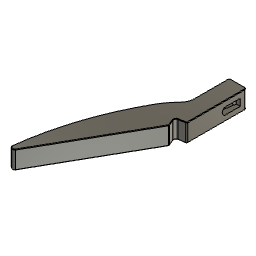
MitiVac Handle v3 (Autodesk Fusion 360 design; units mm, degrees)
Autodesk Fusion 360 part; units mm, degrees
sketch "Sketch1" plane through (0, 0, 0) normal (1, 0, 0) x (0, 1, 0) in component "MitiVac Handle"
  line L0 (0, 0) -> (0, 3.5)
  line L1 (0, 3.5) -> (53.5, 3.5)
  line L2 (53.5, 3.5) -> (53.5, 0)
  line L3 (53.5, 0) -> (37.5, 0)
  line L4 (37.5, 0) -> (35.5, 0)
  line L5 (37.5, 0) -> (37.5, 3.5)
  line L6 (0, 0) -> (0, -3.5)
  line L7 (0, -3.5) -> (53.5, -3.5)
  line L8 (53.5, -3.5) -> (53.5, 0)
  line L9 (37.5, 0) -> (37.5, -3.5)
  arc A0 (37.5, 3.5) -> (37.5, -3.5) centre (39.5625, 0) ccw
  line L10 (0, 0) -> (53.5, 0)
  line L11 (0, 0) -> (53.5, 0)
  line L12 (0, 3.5) -> (0, 9)
  line L13 (0, -3.5) -> (0, -9)
  line L14 (0, 9) -> (30, 9)
  line L15 (30, 9) -> (30, 12.5)
  line L16 (30, 12.5) -> (60, 12.5)
  line L17 (60, 12.5) -> (60, 0)
  line L18 (0, -9) -> (30, -9)
  line L19 (30, -9) -> (30, -12.5)
  line L20 (30, -12.5) -> (60, -12.5)
  line L21 (60, -12.5) -> (60, 0)
  dimension "d1" = 3.5
  dimension "d2" = 53.5
  dimension "d3" = 3.5
  dimension "d4" = 16
  dimension "d5" = 2
  dimension "d6" = 3.5
  dimension "d7" = 53.5
  dimension "d8" = 5.5
  dimension "d9" = 5.5
  dimension "d10" = 30
  dimension "d11" = 3.5
  dimension "d12" = 30
  dimension "d13" = 12.5
  dimension "d14" = 30
  dimension "d15" = 3.5
  dimension "d16" = 30
  constraint coincident L0.start L6.start
  constraint vertical L0
  constraint perpendicular L0 L1
  constraint perpendicular L1 L2
  constraint perpendicular L2 L3
  constraint parallel L3 L4
  constraint coincident L1 L5.end
  constraint perpendicular L1 L5
  constraint parallel L0 L6
  constraint perpendicular L6 L7
  constraint coincident L7 L9.end
  constraint perpendicular L7 L9
  constraint coincident L4.end A0
  constraint perpendicular L1 L12
  constraint perpendicular L7 L13
  constraint perpendicular L12 L14
  constraint perpendicular L14 L15
  constraint perpendicular L15 L16
  constraint perpendicular L16 L17
  constraint perpendicular L13 L18
  constraint perpendicular L18 L19
  constraint perpendicular L19 L20
  measures "d1" distance of L0.start L0.end
  measures "d2" distance of L0.end L1.end
  measures "d3" distance of L1.end L2.end
  measures "d4" distance of L2.end L3.end
  measures "d5" distance of L3.end L4.end
  measures "d6" distance of L0.start L6.end
  measures "d7" distance of L6.end L7.end
  measures "d8" distance of L0.end L12.end
  measures "d9" distance of L6.end L13.end
  measures "d10" distance of L12.end L14.end
  measures "d11" distance of L14.end L15.end
  measures "d12" distance of L15.end L16.end
  measures "d13" distance of L16.end L17.end
  measures "d14" distance of L13.end L18.end
  measures "d15" distance of L18.end L19.end
  measures "d16" distance of L19.end L20.end
sketch "Sketch2" plane through (0, 0, 0) normal (0, 0, 1) x (1, 0, 0) in component "MitiVac Handle"
  line L0 (0, 0) -> (0, 53.5)
  line L1 (0, 0) -> (-10.667, -1.6895)
  line L2 (0, 0) -> (9, 0) construction
  line L3 (-10.667, -1.6895) -> (-6.7597, -10.8945)
  line L4 (-10.667, -1.6895) -> (-0.667, -1.6895) construction
  line L5 (0, 0) -> (-6.7597, -10.8945)
  line L6 (-6.7597, -10.8945) -> (18.2403, -10.8945) construction
  line L7 (0, 0) -> (0, -40)
  line L8 (0, -40) -> (-63.5674, -110.5988)
  line L9 (0, -40) -> (95, -40) construction
  line L10 (-63.5674, -110.5988) -> (-6.7597, -10.8945)
  line L11 (0, 53.5) -> (0, 60)
  line L12 (0, 60) -> (-12.5, 60)
  line L13 (-12.5, 60) -> (-12.5, 25)
  line L14 (-63.5674, -110.5988) -> (-67.9117, -108.1235)
  line L15 (-10.667, -1.6895) -> (-28.7932, 6.7629)
  line L16 (-10.667, -1.6895) -> (9.333, -1.6895) construction
  line L17 (-28.7932, 6.7629) -> (-12.5, 25)
  line L18 (-28.7932, 6.7629) -> (-54.1503, -47.6156)
  arc A0 (-28.7932, 6.7629) -> (-67.9117, -108.1235) centre (217.624, -141.2447) ccw
  line L19 (0, 53.5) -> (-4, 53.5)
  line L20 (0, 53.5) -> (0, 37.5)
  line L21 (0, 37.5) -> (0, 35.5)
  line L22 (0, 37.5) -> (-6.5, 37.5)
  line L23 (-6.5, 37.5) -> (-4, 53.5)
  line L24 (-12.5, 60) -> (-12.5, 56)
  line L25 (-12.5, 56) -> (-4, 53.5)
  line L26 (-6.5, 37.5) -> (-12.5, 37.5)
  line L27 (-12.5, 37.5) -> (-12.5, 35.5)
  line L28 (-6.5, 37.5) -> (-12.5, 35.5)
  line L29 (-12.5, 60) -> (-17.5, 60)
  line L30 (-17.5, 60) -> (-17.5, 19.4035)
  line L31 (-12.5, 35.5) -> (-17.5, 33.8333)
  line L32 (-12.5, 56) -> (-17.5, 57.4706)
  dimension "d17" = 53.5
  dimension "d18" = 10.8
  dimension "d19" = 171
  dimension "d20" = 67
  dimension "d21" = 10
  dimension "d24" = 40
  dimension "d25" = 132
  dimension "d26" = 95
  dimension "d27" = 6.5
  dimension "d28" = 12.5
  dimension "d29" = 35
  dimension "d30" = 5
  dimension "d31" = 155
  dimension "d32" = 20
  dimension "d33" = 60
  dimension "d34" = 4
  dimension "d35" = 16
  dimension "d36" = 2
  dimension "d37" = 6.5
  dimension "d38" = 4
  dimension "d39" = 2
  dimension "d66" = 5
  constraint coincident L0.start L1.start
  constraint vertical L0
  constraint horizontal L2
  constraint horizontal L4
  constraint horizontal L6
  constraint perpendicular L6 L7
  constraint horizontal L9
  constraint parallel L0 L11
  constraint perpendicular L11 L12
  constraint perpendicular L12 L13
  constraint perpendicular L10 L14
  constraint horizontal L16
  constraint perpendicular L15 L18
  constraint coincident L18.end A0
  constraint perpendicular L0 L19
  constraint coincident L0 L20.end
  constraint parallel L0 L21
  constraint perpendicular L20 L22
  constraint perpendicular L19 L24
  constraint coincident L13 L26.end
  constraint perpendicular L13 L26
  constraint perpendicular L26 L27
  constraint perpendicular L24 L29
  constraint coincident L17 L30.end
  constraint perpendicular L29 L30
  constraint coincident L30 L31.end
  constraint parallel L28 L31
  constraint coincident L30 L32.end
  constraint parallel L25 L32
  measures "d17" distance of L0.start L0.end
  measures "d18" distance of L0.start L1.end
  measures "d19" angle of L1 L2
  measures "d20" angle of L3 L4
  measures "d21" distance of L1.end L3.end
  measures "d24" distance of L0.start L7.end
  measures "d25" angle of L8 L9
  measures "d26" distance of L7.end L8.end
  measures "d27" distance of L0.end L11.end
  measures "d28" distance of L11.end L12.end
  measures "d29" distance of L12.end L13.end
  measures "d30" distance of L8.end L14.end
  measures "d31" angle of L15 L16
  measures "d32" distance of L1.end L15.end
  measures "d33" distance of L15.end L18.end
  measures "d34" distance of L0.end L19.end
  measures "d35" distance of L0.end L20.end
  measures "d36" distance of L20.end L21.end
  measures "d37" distance of L20.end L22.end
  measures "d38" distance of L12.end L24.end
  measures "d39" distance of L26.end L27.end
  measures "d66" distance of L12.end L29.end
extrude "Extrude1" add sketch "Sketch2" along normal mid plane 18 contours L0 L1 L13 L15 L17 L21 L22 L28 | L3 L10 L14 L15 L18 A0 | L0 L19 L20 L22 L23 | L18 A0 | L11 L12 L13 L19 L24 L25 | L13 L23 L25 L26 | L13 L26 L27 L28 | L13 L17 L30 L31 | L13 L27 L30 L31 L32 | L13 L24 L29 L30 L32 in component "MitiVac Handle"
extrude "Extrude3" cut sketch "Sketch1" against normal up to surface (17.5 mm away) contours L4 L5 A0 L10 L11 | L4 L9 A0 L10 L11 | L1 L2 L3 L5 L10 L11 | L3 L7 L8 L9 L10 L11 in component "MitiVac Handle"
extrude "Extrude4" cut sketch "Sketch2" along normal mid plane 13.5 contours L13 L23 L25 L26 | L13 L26 L27 L28 | L13 L27 L30 L31 L32 in component "MitiVac Handle"
fillet "Fillet2" radius 2.5 1 edges at (-10.667, -1.6895, 0) in component "MitiVac Handle"
fillet "Fillet2" radius 1 2 edges at (0, 0, 0) (-6.7597, -10.8945, 0) in component "MitiVac Handle"
fillet "Fillet2" radius 2 2 edges at (0, 60, 0) (-17.5, 60, 0) in component "MitiVac Handle"
fillet "Fillet2" radius 12 1 edges at (-17.5, 19.4035, 0) in component "MitiVac Handle"
fillet "Fillet2" radius 65 1 edges at (-28.7932, 6.7629, 0) in component "MitiVac Handle"
fillet "Fillet2" radius 2 2 edges at (-67.9117, -108.1235, 0) (-63.5674, -110.5988, 0) in component "MitiVac Handle"
fillet "Fillet3" radius 0.5 2 faces at (-29.4988, -14.8978, 9) (-29.4988, -14.8978, -9) in component "MitiVac Handle"
component "MitiVac Handle" placed x (1, 0, 0) y (0, 1, 0) z (0, 0, 1) at (0, 0, 0)
equation "d3 = d1"
equation "d6 = d1"
equation "d7 = d2"
equation "d8 = ( 18 / 2 ) * 1 mm - 3.5 mm"
equation "d9 = d8"
equation "d11 = ( 25 / 2 ) * 1 mm - d8 - d1"
equation "d12 = 60 mm - d10"
equation "d13 = d11 + d8 + d1"
equation "d14 = d10"
equation "d15 = d11"
equation "d16 = d12"
equation "d19 = 180 deg - 9 deg"
equation "d25 = 270 deg - 138 deg"
equation "d46 = ( 13.5 / 2 ) * 1 mm"
named bodies: "MitiVac Handle"
